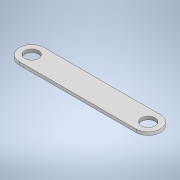
# Autodesk Inventor part: intake-1
Saved by Autodesk Inventor 2022 (Build 260153000, 153)
## iProperties
Created: 2023-01-10
Part Number: intake-1
Material: Generic
Document SubType Name: Modeling
Designer: s135320
Density: 1 g/cm^3
Appearance: Default
Author: s135320
Autodesk Inventor part; units mm, degrees
ref_plane "YZ Plane" through (0, 0, 0) normal (1, 0, 0) x (0, 1, 0)
ref_plane "XZ Plane" through (0, 0, 0) normal (0, 1, 0) x (-1, 0, 0)
ref_plane "XY Plane" through (0, 0, 0) normal (0, 0, 1) x (1, 0, 0)
sketch "Sketch1" plane through (0, 0, 0) normal (0, 1, 0) x (-1, 0, 0)
  line L0 (0, 0) -> (241.3, 0)
  line L1 (0, -25.4) -> (241.3, -25.4)
  line L2 (0, 25.4) -> (241.3, 25.4)
  circle A0 centre (241.3, 0) radius 25.4
  circle A1 centre (0, 0) radius 25.4
  circle A2 centre (241.3, 0) radius 14.2875
  circle A3 centre (0, 0) radius 14.2875
  dimension "d0" = 25.4
  dimension "d1" = 25.4
  dimension "d2" = 28.575
  dimension "d3" = 28.575
  dimension "d6" = 241.3
  constraints: 6 end point, 4 centre point, 4 coincident, 4 point on circle, 2 parallel, 2 tangent, 1 horizontal
  measures "d0" distance between parallel lines of L0 L2
  measures "d1" distance between parallel lines of L1 L0
  measures "d2" diameter of A3
  measures "d3" diameter of A2
  measures "d6" distance of L0.start L0.end
extrude "Extrusion1" add sketch "Sketch1" along normal blind 6.35
equation "\"d0\" = d1"
body "Solid1"
